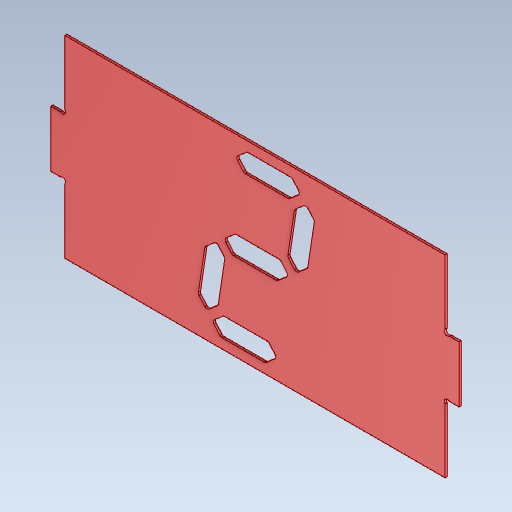
# Autodesk Inventor part: Cockpit_front_frame_cloth
Saved by Autodesk Inventor 2020 (Build 240168000, 168)
## iProperties
Created: 2022-04-24
Part Number: Cockpit_front_frame_cloth
Material: PET プラスチック
Document SubType Name: Modeling
Designer: Masato Kubotera
Density: 1.541 g/cm^3
Appearance: 滑らか - 赤
Description: PP T0.75
Author: Masato Kubotera
Autodesk Inventor part; units mm, degrees
ref_plane "YZ Plane" through (0, 0, 0) normal (1, 0, 0) x (0, 1, 0)
ref_plane "XZ Plane" through (0, 0, 0) normal (0, 1, 0) x (-1, 0, 0)
ref_plane "XY Plane" through (0, 0, 0) normal (0, 0, 1) x (1, 0, 0)
derived "Cockpit_front_frame.ipt"
sketch "スケッチ2" plane through (0, 0, 0) normal (0, 1, 0) x (-1, 0, 0)
  line L0 (-23.5, -22.5) -> (-28.5, -27.5)
  line L1 (-28.5, -27.5) -> (-28.5, -91)
  line L2 (-28.5, -91) -> (-23.5, -96)
  line L3 (-23.5, -96) -> (35.75, -96)
  line L4 (37.75, -98) -> (37.75, -131)
  line L5 (37.75, -131) -> (42.75, -136)
  line L6 (42.75, -136) -> (83.5, -136)
  line L7 (88.5, -131) -> (88.5, -20)
  line L8 (88.5, -20) -> (86, -17.5)
  line L9 (86, -17.5) -> (80.25, -17.5)
  line L10 (80.25, -17.5) -> (80.25, -22.5)
  line L11 (80.25, -22.5) -> (73.9849, -22.5)
  line L12 (72.5, -21.0151) -> (72.5, -17.5)
  line L13 (72.5, -17.5) -> (64.5, -17.5)
  line L14 (64.5, -17.5) -> (64.5, -21.0151)
  line L15 (63.0151, -22.5) -> (-23.5, -22.5)
  line L16 (-25.25, -25) -> (-20.25, -25) construction
  line L17 (-20.25, -25) -> (-20.25, -93.5) construction
  line L18 (-20.25, -93.5) -> (-25.25, -93.5) construction
  line L19 (-25.25, -93.5) -> (-25.25, -25) construction
  line L20 (-26, -25) -> (-25.25, -25) construction
  line L21 (-25.25, -93.5) -> (-26, -93.5) construction
  line L22 (-26, -93.5) -> (-26, -25) construction
  line L23 (-20.25, -93.5) -> (80.25, -93.5) construction
  line L24 (-20.25, -88.5) -> (80.25, -88.5) construction
  line L25 (80.25, -22.5) -> (80.25, -90.5) construction
  line L26 (80.25, -90.5) -> (85.25, -90.5) construction
  line L27 (85.25, -90.5) -> (85.25, -22.5) construction
  line L28 (80.25, -88.5) -> (80.25, -93.5) construction
  line L29 (80.25, -91) -> (85.25, -91) construction
  line L30 (85.25, -91) -> (85.25, -133.5) construction
  line L31 (80.25, -91) -> (80.25, -133.5) construction
  line L32 (80.25, -133.5) -> (85.25, -133.5) construction
  line L33 (40.25, -133.5) -> (40.25, -128.5) construction
  line L34 (40.25, -128.5) -> (40.25, -93.5) construction
  line L35 (45.25, -93.5) -> (45.25, -128.5) construction
  line L36 (40.25, -128.5) -> (45.25, -128.5) construction
  line L37 (42.75, -128.5) -> (42.75, -93.5) construction
  line L38 (40.25, -128.5) -> (79.1145, -128.5) construction
  line L39 (79.1145, -128.5) -> (79.1145, -133.5) construction
  line L40 (79.1145, -133.5) -> (40.25, -133.5) construction
  line L41 (40.25, -131) -> (79.1145, -131) construction
  line L42 (82.75, -91) -> (82.75, -133.5) construction
  circle A0 centre (82.75, -131) radius 2
  arc A1 (80.25, -128.5) -> (85.25, -128.5) centre (82.75, -131) ccw construction
  line L43 (80.25, -91) -> (-20.25, -91) construction
  line L44 (42.75, -111) -> (45.25, -111) construction
  line L45 (59.6822, -128.5) -> (59.6822, -131) construction
  line L46 (42.7, -115.5651) -> (42.7, -106.4349)
  line L47 (45.3, -107.05) -> (45.3, -114.95)
  line L48 (45.3, -117.05) -> (42.7, -104.95) construction
  line L49 (42.7, -117.05) -> (45.3, -104.95) construction
  line L50 (55.7322, -128.45) -> (63.6322, -128.45)
  line L51 (64.2473, -131.05) -> (55.1172, -131.05)
  line L52 (53.6322, -128.45) -> (65.7322, -131.05) construction
  line L53 (65.7322, -128.45) -> (53.6322, -131.05) construction
  line L54 (42.75, -105) -> (45.25, -105) construction
  line L55 (42.75, -117) -> (45.25, -117) construction
  arc A2 (44.1849, -104.95) -> (42.7, -106.4349) centre (43.4425, -105.6925) ccw
  arc A3 (45.3, -107.05) -> (45.3, -104.95) centre (45.3, -106) ccw
  arc A4 (42.7, -115.5651) -> (44.1849, -117.05) centre (43.4425, -116.3075) ccw
  arc A5 (45.3, -117.05) -> (45.3, -114.95) centre (45.3, -116) ccw
  line L56 (53.6822, -131) -> (53.6822, -128.5) construction
  line L57 (65.6822, -128.5) -> (65.6822, -131) construction
  arc A6 (53.6322, -129.5651) -> (55.1172, -131.05) centre (54.3747, -130.3075) ccw
  arc A7 (55.7322, -128.45) -> (53.6322, -128.45) centre (54.6822, -128.45) ccw
  arc A8 (64.2473, -131.05) -> (65.7322, -129.5651) centre (64.9898, -130.3075) ccw
  arc A9 (65.7322, -128.45) -> (63.6322, -128.45) centre (64.6822, -128.45) ccw
  line L58 (53.6322, -129.5651) -> (53.6322, -128.45)
  line L59 (65.7322, -128.45) -> (65.7322, -129.5651)
  line L60 (44.1849, -104.95) -> (45.3, -104.95)
  line L61 (45.3, -117.05) -> (44.1849, -117.05)
  circle A10 centre (47.6822, -131) radius 1.6
  line L62 (85.25, -22.5) -> (85.25, -17.5) construction
  line L63 (86, -17.5) -> (86, -90.5) construction
  line L64 (86, -90.5) -> (85.25, -90.5) construction
  line L65 (-18.5, -82.5) -> (-18.5, -61)
  arc A11 (-18.5, -82.5) -> (-16.5, -84.5) centre (-16.5, -82.5) ccw
  line L66 (45.5, -84.5) -> (-16.5, -84.5)
  arc A12 (45.5, -84.5) -> (47.5, -82.5) centre (45.5, -82.5) ccw
  line L67 (47.5, -61) -> (47.5, -82.5)
  arc A13 (47.5, -61) -> (45.5, -59) centre (45.5, -61) ccw
  line L68 (-16.5, -59) -> (45.5, -59)
  arc A14 (-16.5, -59) -> (-18.5, -61) centre (-16.5, -61) ccw
  line L69 (30, -88.5) -> (30, -91) construction
  line L70 (82.75, -22.5) -> (82.75, -90.5) construction
  circle A15 centre (82.75, -34) radius 1.6
  circle A16 centre (82.75, -34) radius 3
  circle A17 centre (82.75, -79) radius 1.6
  circle A18 centre (82.75, -79) radius 3
  line L71 (85.25, -22.5) -> (80.25, -22.5) construction
  arc A19 (85.25, -91) -> (80.25, -91) centre (82.75, -131) ccw construction
  circle A20 centre (47.6822, -131) radius 3
  circle A21 centre (42.75, -99) radius 1.6
  circle A22 centre (42.75, -99) radius 3
  line L72 (5, -88.5) -> (5, -91) construction
  line L73 (55, -88.5) -> (55, -91) construction
  line L74 (53.5651, -91.05) -> (6.4349, -91.05)
  line L75 (4.95, -89.5651) -> (4.95, -88.45)
  line L76 (7.05, -88.45) -> (52.95, -88.45)
  line L77 (55.05, -88.45) -> (55.05, -89.5651)
  line L78 (55.05, -91.05) -> (4.95, -88.45) construction
  line L79 (4.95, -91.05) -> (55.05, -88.45) construction
  arc A23 (7.05, -88.45) -> (4.95, -88.45) centre (6, -88.45) ccw
  arc A24 (4.95, -89.5651) -> (6.4349, -91.05) centre (5.6925, -90.3075) ccw
  arc A25 (55.05, -88.45) -> (52.95, -88.45) centre (54, -88.45) ccw
  arc A26 (53.5651, -91.05) -> (55.05, -89.5651) centre (54.3075, -90.3075) ccw
  line L80 (-20.25, -41) -> (80.25, -41) construction
  line L81 (80.25, -36) -> (-20.25, -36) construction
  line L82 (-20.25, -36) -> (-20.25, -41) construction
  line L83 (-20.25, -38.5) -> (80.25, -38.5) construction
  line L84 (30, -41) -> (30, -36) construction
  line L85 (53.5651, -35.95) -> (6.4349, -35.95)
  line L86 (6.4349, -41.05) -> (53.5651, -41.05)
  line L87 (55.05, -35.95) -> (4.95, -41.05) construction
  line L88 (4.95, -35.95) -> (55.5723, -41.1032) construction
  arc A27 (6.4349, -35.95) -> (4.95, -37.4349) centre (5.6925, -36.6925) ccw
  arc A28 (4.95, -39.5651) -> (6.4349, -41.05) centre (5.6925, -40.3075) ccw
  arc A29 (55.05, -37.4349) -> (53.5651, -35.95) centre (54.3075, -36.6925) ccw
  arc A30 (53.5651, -41.05) -> (55.05, -39.5651) centre (54.3075, -40.3075) ccw
  line L89 (5, -41) -> (5, -36) construction
  line L90 (55, -36) -> (55, -41) construction
  line L91 (4.95, -37.4349) -> (4.95, -39.5651)
  line L92 (55.05, -39.5651) -> (55.05, -37.4349)
  circle A31 centre (-2.5, -38.5) radius 1.6
  circle A32 centre (-2.5, -38.5) radius 3
  circle A33 centre (62.5, -38.5) radius 1.6
  circle A34 centre (62.5, -38.5) radius 3
  line L93 (-25.25, -44.25) -> (-22.75, -44.25) construction
  line L94 (-25.25, -49.25) -> (-26, -49.25) construction
  line L95 (-25.25, -74.25) -> (-22.75, -74.25) construction
  line L96 (-25.25, -69.25) -> (-26, -69.25) construction
  line L97 (-26, -59.25) -> (-25.25, -59.25) construction
  line L98 (-25.25, -59.25) -> (-22.75, -59.25) construction
  line L99 (-22.75, -25) -> (-22.75, -93.5) construction
  arc A35 (63.0151, -22.5) -> (64.5, -21.0151) centre (63.7575, -21.7575) ccw
  arc A36 (72.5, -21.0151) -> (73.9849, -22.5) centre (73.2425, -21.7575) ccw
  line L100 (56.75, -22.5) -> (56.75, -32.5) construction
  line L101 (56.75, -32.5) -> (80.25, -32.5) construction
  line L102 (80.25, -32.5) -> (80.25, -22.5) construction
  line L103 (68.5, -17.5) -> (68.5, -32.5) construction
  line L104 (60.5, -22.5) -> (60.5, -17.5) construction
  line L105 (76.5, -22.5) -> (76.5, -17.5) construction
  line L106 (-22.7, -46.3) -> (-22.7, -72.2)
  line L107 (-25.3, -72.8151) -> (-25.3, -69.564)
  line L108 (-25.3, -44.2) -> (-22.7, -74.3) construction
  line L109 (-22.7, -44.2) -> (-25.3, -74.3) construction
  arc A37 (-22.7, -46.3) -> (-22.7, -44.2) centre (-22.7, -45.25) ccw
  arc A38 (-23.8151, -44.2) -> (-25.3, -45.6849) centre (-24.5575, -44.9425) ccw
  line L110 (-23.8151, -44.2) -> (-22.7, -44.2)
  arc A39 (-22.7, -74.3) -> (-22.7, -72.2) centre (-22.7, -73.25) ccw
  arc A40 (-25.3, -72.8151) -> (-23.8151, -74.3) centre (-24.5575, -73.5575) ccw
  line L111 (-22.7, -74.3) -> (-23.8151, -74.3)
  line L112 (-26.3, -49.9848) -> (-26.3, -68.5152)
  arc A41 (-26.3, -68.5152) -> (-25.3, -69.564) centre (-25.25, -68.5152) ccw
  arc A42 (-25.3, -48.936) -> (-26.3, -49.9848) centre (-25.25, -49.9848) ccw
  line L113 (-25.3, -48.936) -> (-25.3, -45.6849)
  circle A43 centre (-22.75, -36.75) radius 1.6
  circle A44 centre (-22.75, -36.75) radius 3
  circle A45 centre (-22.75, -81.75) radius 1.6
  circle A46 centre (-22.75, -81.75) radius 3
  line L114 (64.5, -22.5) -> (72.5, -22.5)
  line L115 (85.25, -17.5) -> (52.5, -17.5) construction
  line L116 (52.5, -17.5) -> (52.5, -22.5) construction
  circle A47 centre (82.75, -93.5) radius 1.475
  circle A48 centre (82.75, -98.5) radius 1.475
  circle A49 centre (82.75, -103.5) radius 1.475
  line L117 (49.75, -93.5) -> (78.25, -93.5)
  line L118 (80.25, -95.5) -> (80.25, -124)
  line L119 (78.25, -126) -> (49.75, -126)
  line L120 (47.75, -124) -> (47.75, -95.5)
  arc A50 (49.75, -93.5) -> (47.75, -95.5) centre (49.75, -95.5) ccw
  arc A51 (47.75, -124) -> (49.75, -126) centre (49.75, -124) ccw
  arc A52 (78.25, -126) -> (80.25, -124) centre (78.25, -124) ccw
  arc A53 (80.25, -95.5) -> (78.25, -93.5) centre (78.25, -95.5) ccw
  arc A54 (37.75, -98) -> (35.75, -96) centre (35.75, -98) ccw
  circle A55 centre (-13.5, -55) radius 1.75
  circle A56 centre (-13.5, -55) radius 2
  line L121 (74.85, -78.65) -> (65.65, -78.65) construction
  line L122 (65.65, -78.65) -> (65.65, -64.85) construction
  line L123 (65.65, -64.85) -> (74.85, -64.85) construction
  line L124 (74.85, -64.85) -> (74.85, -78.65) construction
  line L125 (74.85, -78.65) -> (65.65, -64.85) construction
  line L126 (65.65, -78.65) -> (74.85, -64.85) construction
  line L127 (64.95, -64.2) -> (75.55, -64.2) construction
  line L128 (75.55, -64.2) -> (75.55, -79.3) construction
  line L129 (75.55, -79.3) -> (64.95, -79.3) construction
  line L130 (64.95, -79.3) -> (64.95, -64.2) construction
  line L131 (64.95, -64.2) -> (75.55, -79.3) construction
  line L132 (75.55, -64.2) -> (64.95, -79.3) construction
  line L133 (66.3849, -64.15) -> (74.1151, -64.15)
  line L134 (75.6, -65.6349) -> (75.6, -77.8651)
  line L135 (75.6, -79.35) -> (64.9, -64.15) construction
  line L136 (64.9, -79.35) -> (75.6, -64.15) construction
  line L137 (74.9, -78.7) -> (65.6, -64.8) construction
  line L138 (65.6, -78.7) -> (74.9, -64.8) construction
  arc A57 (66.3849, -64.15) -> (64.9, -65.6349) centre (65.6425, -64.8925) ccw
  arc A58 (67.0849, -64.8) -> (65.6, -66.2849) centre (66.3425, -65.5425) ccw
  line L139 (64.9, -71.75) -> (75.6, -71.75) construction
  line L140 (70.25, -64.15) -> (70.25, -78.7063) construction
  arc A59 (75.6, -65.6349) -> (74.1151, -64.15) centre (74.8575, -64.8925) ccw
  arc A60 (74.9, -66.2849) -> (73.4151, -64.8) centre (74.1575, -65.5425) ccw
  arc A61 (64.9, -77.8651) -> (66.3849, -79.35) centre (65.6425, -78.6075) ccw
  arc A62 (65.6, -77.2151) -> (67.0849, -78.7) centre (66.3425, -77.9575) ccw
  arc A63 (74.1151, -79.35) -> (75.6, -77.8651) centre (74.8575, -78.6075) ccw
  arc A64 (73.4151, -78.7) -> (74.9, -77.2151) centre (74.1575, -77.9575) ccw
  line L141 (67.0849, -64.8) -> (73.4151, -64.8)
  line L142 (74.9, -66.2849) -> (74.9, -77.2151)
  line L143 (64.9, -77.8651) -> (64.9, -65.6349)
  line L144 (65.6, -77.2151) -> (65.6, -66.2849)
  line L145 (73.4151, -78.7) -> (67.0849, -78.7)
  line L146 (74.1151, -79.35) -> (66.3849, -79.35)
  line L147 (-18.5, -71.75) -> (47.5, -71.75) construction
  line L148 (82.75, -56.5) -> (85.25, -56.5) construction
  line L149 (86, -54) -> (85.25, -54) construction
  line L150 (82.7, -69.45) -> (82.7, -43.55)
  line L151 (85.3057, -71.616) -> (82.7, -41.45) construction
  line L152 (82.7, -71.55) -> (85.3, -41.45) construction
  arc A65 (82.7, -41.45) -> (82.7, -43.55) centre (82.7, -42.5) ccw
  arc A66 (85.3, -42.9349) -> (83.8151, -41.45) centre (84.5575, -42.1925) ccw
  arc A67 (82.7, -69.45) -> (82.7, -71.55) centre (82.7, -70.5) ccw
  arc A68 (83.8151, -71.55) -> (85.3, -70.0651) centre (84.5575, -70.8075) ccw
  line L153 (82.75, -41.5) -> (85.25, -41.5) construction
  line L154 (82.75, -71.5) -> (85.25, -71.5) construction
  arc A69 (86.25, -47.1801) -> (85.3, -46.1348) centre (85.2, -47.1801) ccw
  line L155 (86.25, -47.1801) -> (86.25, -65.8199)
  line L156 (85.25, -46.5) -> (86, -46.5) construction
  line L157 (85.25, -66.5) -> (86, -66.5) construction
  arc A70 (85.3, -66.8652) -> (86.25, -65.8199) centre (85.2, -65.8199) ccw
  line L158 (85.3, -42.9349) -> (85.3, -46.1348)
  line L159 (85.3, -66.8652) -> (85.3, -70.0651)
  line L160 (83.8151, -71.55) -> (82.7, -71.55)
  line L161 (82.7, -41.45) -> (83.8151, -41.45)
  line L162 (83.5, -136) -> (88.5, -131)
  point P0 (0, 0)
  point P1 (-25.7227, -96)
  point P2 (-23.5, -22.5)
  point P3 (44, -111)
  point P4 (59.6822, -129.75)
  point P5 (30, -89.75)
  point P6 (30, -38.5)
  point P7 (4.95, -41.05)
  point P8 (52.5, -22)
  point P9 (-24, -59.25)
  point P10 (70.25, -71.75)
  point P11 (70.25, -71.75)
  point P12 (84, -56.5)
  dimension "d4" = 0.75
  measures "d4" distance of L20.start L20.end
sketch "スケッチ3" plane through (25.25, 0, 0) normal (1, 0, 0) x (0, 1, 0)
  line L0 (-135, -25) -> (0, -25)
  line L1 (0, -93.5) -> (-135, -93.5)
  line L2 (1.4849, -44.25) -> (5, -44.25)
  line L3 (5, -44.25) -> (5, -74.25)
  line L4 (0, -59.25) -> (-135, -59.25) construction
  arc A0 (0, -42.7651) -> (1.4849, -44.25) centre (0.7425, -43.5075) ccw
  line L5 (0, -25) -> (0, -42.7651)
  arc A1 (1.4849, -74.25) -> (0, -75.7349) centre (0.7425, -74.9925) ccw
  line L6 (1.4849, -74.25) -> (5, -74.25)
  line L7 (0, -44.25) -> (0, -74.25)
  line L8 (0, -75.7349) -> (0, -93.5)
  line L9 (-67.5, -25) -> (-67.5, -93.5) construction
  line L10 (-136.4849, -74.25) -> (-140, -74.25)
  arc A2 (-135, -75.7349) -> (-136.4849, -74.25) centre (-135.7425, -74.9925) ccw
  line L11 (-136.4849, -44.25) -> (-140, -44.25)
  line L12 (-140, -44.25) -> (-140, -74.25)
  line L13 (-135, -75.7349) -> (-135, -93.5)
  arc A3 (-136.4849, -44.25) -> (-135, -42.7651) centre (-135.7425, -43.5075) ccw
  line L14 (-135, -44.25) -> (-135, -74.25)
  line L15 (-135, -25) -> (-135, -42.7651)
  line L16 (-7, -30) -> (-128, -30)
  line L17 (-130, -32) -> (-130, -34)
  line L18 (-128, -36) -> (-7, -36)
  line L19 (-5, -34) -> (-5, -32)
  line L20 (-5, -30) -> (-130, -36) construction
  line L21 (-130, -30) -> (-5, -36) construction
  line L22 (-7, -88.5) -> (-128, -88.5)
  line L23 (-130, -86.5) -> (-130, -43)
  line L24 (-128, -41) -> (-7, -41)
  line L25 (-5, -43) -> (-5, -86.5)
  line L26 (-5, -88.5) -> (-130, -41) construction
  line L27 (-130, -88.5) -> (-5, -41) construction
  arc A4 (-128, -30) -> (-130, -32) centre (-128, -32) ccw
  arc A5 (-130, -34) -> (-128, -36) centre (-128, -34) ccw
  arc A6 (-7, -36) -> (-5, -34) centre (-7, -34) ccw
  arc A7 (-5, -32) -> (-7, -30) centre (-7, -32) ccw
  arc A8 (-5, -43) -> (-7, -41) centre (-7, -43) ccw
  arc A9 (-128, -41) -> (-130, -43) centre (-128, -43) ccw
  arc A10 (-130, -86.5) -> (-128, -88.5) centre (-128, -86.5) ccw
  arc A11 (-7, -88.5) -> (-5, -86.5) centre (-7, -86.5) ccw
  point P0 (0, 0)
  point P1 (0, -93.5)
  point P2 (-135, -93.5)
  point P3 (-135, -25)
  point P4 (-67.5, -33)
  point P5 (-67.5, -64.75)
  point P6 (0, -36)
  point P7 (0, -36)
  point P8 (0, -36)
  point P9 (0, -41)
  point P10 (0, -41)
  point P11 (0, -41)
ref_plane "作業平面1" through (25.25, -135, -25) normal (-1, 0, 0) x (0, 1, 0)
sketch "スケッチ4" plane through (25.25, -135, -25) normal (-1, 0, 0) x (0, 1, 0)
  arc A0 (136.4849, 24.25) -> (135, 22.7651) centre (135.7425, 23.5075) ccw
  line L0 (136.4849, 24.25) -> (140, 24.25)
  line L1 (140, 24.25) -> (140, 44.25)
  line L2 (135, 19.25) -> (135, 49.25) construction
  line L3 (140, 19.25) -> (140, 49.25) construction
  line L4 (135, 34.25) -> (0, 34.25) construction
  line L5 (67.5, 0) -> (67.5, 68.5) construction
  line L6 (0, 0) -> (135, 0) projected
  line L7 (135, 68.5) -> (0, 68.5) projected
  arc A1 (135, 45.7349) -> (136.4849, 44.25) centre (135.7425, 44.9925) ccw
  line L8 (136.4849, 44.25) -> (140, 44.25)
  line L9 (135, 22.7651) -> (135, 0)
  line L10 (135, 45.7349) -> (135, 68.5)
  arc A2 (0, 22.7651) -> (-1.4849, 24.25) centre (-0.7425, 23.5075) ccw
  line L11 (-1.4849, 24.25) -> (-5, 24.25)
  line L12 (-1.4849, 44.25) -> (-5, 44.25)
  arc A3 (-1.4849, 44.25) -> (0, 45.7349) centre (-0.7425, 44.9925) ccw
  line L13 (0, 22.7651) -> (0, 0)
  line L14 (0, 45.7349) -> (0, 68.5)
  line L15 (-5, 24.25) -> (-5, 44.25)
  line L16 (51.1141, 58.6095) -> (54.1517, 56.0021)
  line L17 (53.0682, 60.8859) -> (56.1057, 58.2784)
  line L18 (55.0145, 64.6885) -> (52.9607, 62.296)
  line L19 (49.704, 58.5021) -> (47.6502, 56.1095)
  line L20 (55.7733, 65.0372) -> (70.8617, 65.0372)
  line L21 (72.6043, 58.3859) -> (74.658, 60.7784)
  line L22 (71.513, 64.796) -> (74.5506, 62.1885)
  line L23 (56.7571, 58.0372) -> (71.8455, 58.0372)
  line L24 (54.4888, 55.3948) -> (56.7748, 40.4805)
  line L25 (56.5452, 39.6777) -> (54.4914, 37.2851)
  line L26 (53.0813, 37.1777) -> (50.0437, 39.7851)
  line L27 (47.4206, 55.3066) -> (49.7066, 40.3924)
  line L28 (50.3553, 59.2608) -> (53.84, 36.5264) construction
  line L29 (75.3094, 61.5372) -> (52.3094, 61.5372) construction
  arc A4 (51.1141, 58.6095) -> (49.704, 58.5021) centre (50.4628, 57.8507) ccw
  arc A5 (54.4888, 55.3948) -> (54.1517, 56.0021) centre (53.5003, 55.2433) ccw
  arc A6 (56.5452, 39.6777) -> (56.7748, 40.4805) centre (55.7864, 40.329) ccw
  arc A7 (53.0813, 37.1777) -> (54.4914, 37.2851) centre (53.7326, 37.9365) ccw
  arc A8 (49.7066, 40.3924) -> (50.0437, 39.7851) centre (50.695, 40.5439) ccw
  arc A9 (47.6502, 56.1095) -> (47.4206, 55.3066) centre (48.409, 55.4582) ccw
  arc A10 (71.8455, 58.0372) -> (72.6043, 58.3859) centre (71.8455, 59.0372) ccw
  arc A11 (74.658, 60.7784) -> (74.5506, 62.1885) centre (73.8992, 61.4298) ccw
  arc A12 (71.513, 64.796) -> (70.8617, 65.0372) centre (70.8617, 64.0372) ccw
  arc A13 (55.7733, 65.0372) -> (55.0145, 64.6885) centre (55.7733, 64.0372) ccw
  arc A14 (52.9607, 62.296) -> (53.0682, 60.8859) centre (53.7195, 61.6446) ccw
  arc A15 (56.1057, 58.2784) -> (56.7571, 58.0372) centre (56.7571, 59.0372) ccw
  line L30 (78.72, 58.6095) -> (81.7576, 56.0021)
  line L31 (77.3099, 58.5021) -> (75.2561, 56.1095)
  arc A16 (78.72, 58.6095) -> (77.3099, 58.5021) centre (78.0687, 57.8507) ccw
  line L32 (75.0264, 55.3066) -> (77.3125, 40.3924)
  arc A17 (75.2561, 56.1095) -> (75.0264, 55.3066) centre (76.0149, 55.4582) ccw
  arc A18 (82.0947, 55.3948) -> (81.7576, 56.0021) centre (81.1062, 55.2433) ccw
  line L33 (82.0947, 55.3948) -> (84.3807, 40.4805)
  arc A19 (84.151, 39.6777) -> (84.3807, 40.4805) centre (83.3922, 40.329) ccw
  line L34 (84.151, 39.6777) -> (82.0973, 37.2851)
  arc A20 (80.6871, 37.1777) -> (82.0973, 37.2851) centre (81.3385, 37.9365) ccw
  line L35 (80.6871, 37.1777) -> (77.6496, 39.7851)
  arc A21 (77.3125, 40.3924) -> (77.6496, 39.7851) centre (78.3009, 40.5439) ccw
  line L36 (55.2967, 31.3223) -> (58.3342, 28.7149)
  line L37 (53.8865, 31.2149) -> (51.8328, 28.8223)
  arc A22 (55.2967, 31.3223) -> (53.8865, 31.2149) centre (54.6453, 30.5635) ccw
  line L38 (51.6031, 28.0195) -> (53.8891, 13.1052)
  arc A23 (51.8328, 28.8223) -> (51.6031, 28.0195) centre (52.5915, 28.171) ccw
  arc A24 (58.6713, 28.1076) -> (58.3342, 28.7149) centre (57.6829, 27.9561) ccw
  line L39 (58.6713, 28.1076) -> (60.9573, 13.1934)
  arc A25 (60.7277, 12.3905) -> (60.9573, 13.1934) centre (59.9689, 13.0418) ccw
  line L40 (60.7277, 12.3905) -> (58.6739, 9.9979)
  arc A26 (57.2638, 9.8905) -> (58.6739, 9.9979) centre (57.9151, 10.6493) ccw
  line L41 (57.2638, 9.8905) -> (54.2262, 12.4979)
  arc A27 (53.8891, 13.1052) -> (54.2262, 12.4979) centre (54.8776, 13.2567) ccw
  line L42 (82.9025, 31.3223) -> (85.9401, 28.7149)
  line L43 (81.4924, 31.2149) -> (79.4386, 28.8223)
  arc A28 (82.9025, 31.3223) -> (81.4924, 31.2149) centre (82.2512, 30.5635) ccw
  line L44 (79.209, 28.0195) -> (81.495, 13.1052)
  arc A29 (79.4386, 28.8223) -> (79.209, 28.0195) centre (80.1974, 28.171) ccw
  arc A30 (86.2772, 28.1076) -> (85.9401, 28.7149) centre (85.2887, 27.9561) ccw
  line L45 (86.2772, 28.1076) -> (88.5632, 13.1934)
  arc A31 (88.3336, 12.3905) -> (88.5632, 13.1934) centre (87.5748, 13.0418) ccw
  line L46 (88.3336, 12.3905) -> (86.2798, 9.9979)
  arc A32 (84.8697, 9.8905) -> (86.2798, 9.9979) centre (85.521, 10.6493) ccw
  line L47 (84.8697, 9.8905) -> (81.8321, 12.4979)
  arc A33 (81.495, 13.1052) -> (81.8321, 12.4979) centre (82.4834, 13.2567) ccw
  line L48 (59.9558, 37.75) -> (75.0442, 37.75)
  arc A34 (59.9558, 37.75) -> (59.197, 37.4013) centre (59.9558, 36.75) ccw
  line L49 (59.197, 37.4013) -> (57.1432, 35.0088)
  arc A35 (57.1432, 35.0088) -> (57.2507, 33.5987) centre (57.902, 34.3574) ccw
  line L50 (57.2507, 33.5987) -> (60.2882, 30.9912)
  arc A36 (60.2882, 30.9912) -> (60.9396, 30.75) centre (60.9396, 31.75) ccw
  line L51 (60.9396, 30.75) -> (76.028, 30.75)
  arc A37 (76.028, 30.75) -> (76.7868, 31.0987) centre (76.028, 31.75) ccw
  line L52 (76.7868, 31.0987) -> (78.8406, 33.4912)
  arc A38 (78.8406, 33.4912) -> (78.7331, 34.9013) centre (78.0818, 34.1426) ccw
  line L53 (75.6955, 37.5088) -> (78.7331, 34.9013)
  arc A39 (75.6955, 37.5088) -> (75.0442, 37.75) centre (75.0442, 36.75) ccw
  line L54 (64.1383, 10.4628) -> (79.2267, 10.4628)
  arc A40 (64.1383, 10.4628) -> (63.3795, 10.1141) centre (64.1383, 9.4628) ccw
  line L55 (63.3795, 10.1141) -> (61.3258, 7.7216)
  arc A41 (61.3258, 7.7216) -> (61.4332, 6.3115) centre (62.0845, 7.0702) ccw
  line L56 (61.4332, 6.3115) -> (64.4708, 3.704)
  arc A42 (64.4708, 3.704) -> (65.1221, 3.4628) centre (65.1221, 4.4628) ccw
  line L57 (65.1221, 3.4628) -> (80.2105, 3.4628)
  arc A43 (80.2105, 3.4628) -> (80.9693, 3.8115) centre (80.2105, 4.4628) ccw
  line L58 (80.9693, 3.8115) -> (83.0231, 6.204)
  arc A44 (83.0231, 6.204) -> (82.9156, 7.6141) centre (82.2643, 6.8554) ccw
  line L59 (79.8781, 10.2216) -> (82.9156, 7.6141)
  arc A45 (79.8781, 10.2216) -> (79.2267, 10.4628) centre (79.2267, 9.4628) ccw
  line L60 (67.5, 37.75) -> (68.4838, 30.75) construction
  point P0 (135, -25)
  point P1 (135, 24.25)
  point P2 (135, 24.25)
  point P3 (135, 24.25)
  point P4 (135, 24.25)
  point P5 (47.3509, 55.7608)
  point P6 (54.4327, 55.7608)
  point P7 (56.3867, 58.0372)
  point P8 (55.3138, 65.0372)
  point P9 (71.232, 65.0372)
  point P10 (72.305, 58.0372)
  point P11 (56.8444, 40.0264)
  point P12 (49.7627, 40.0264)
  point P13 (77.9612, 59.2608)
  point P14 (82.0386, 55.7608)
  point P15 (74.9568, 55.7608)
  point P16 (77.3686, 40.0264)
  point P17 (84.4503, 40.0264)
  point P18 (81.4459, 36.5264)
  point P19 (54.5379, 31.9736)
  point P20 (58.6152, 28.4736)
  point P21 (51.5335, 28.4736)
  point P22 (53.9452, 12.7392)
  point P23 (61.027, 12.7392)
  point P24 (58.0226, 9.2392)
  point P25 (82.1437, 31.9736)
  point P26 (86.2211, 28.4736)
  point P27 (79.1393, 28.4736)
  point P28 (81.5511, 12.7392)
  point P29 (88.6328, 12.7392)
  point P30 (85.6284, 9.2392)
  point P31 (75.4145, 37.75)
  point P32 (59.4963, 37.75)
  point P33 (56.4919, 34.25)
  point P34 (60.5692, 30.75)
  point P35 (76.4875, 30.75)
  point P36 (79.4919, 34.25)
  point P37 (79.5971, 10.4628)
  point P38 (63.6788, 10.4628)
  point P39 (60.6744, 6.9628)
  point P40 (64.7518, 3.4628)
  point P41 (80.67, 3.4628)
  point P42 (83.6744, 6.9628)
  dimension "d1" = 1.05
  dimension "d13" = 3
  dimension "d14" = 7
  dimension "d15" = 7
  dimension "d16" = 23
  dimension "d17" = 23
  dimension "d18" = 1
  dimension "d19" = 1
  dimension "d20" = 27.6059
  dimension "d21" = 27.6059
  dimension "d22" = 27.6059
  dimension "d25" = 8
  constraints: 110 end point, 93 point on circle, 89 point on line, 46 centre point, 24 tangent, 12 symmetric about line, 10 equal radius, 7 collinear, 6 parallel, 2 horizontal, 2 midpoint, 2 perpendicular, 1 vertical, 190 other
  measures "d1" radius of A0
  measures "d13" distance between parallel lines of L16 L17
  measures "d14" distance between parallel lines of L23 L20
  measures "d15" distance between parallel lines of L24 L27
  measures "d16" distance of L29.start L29.end
  measures "d17" distance of L28.start L28.end
  measures "d18" radius of A4
  measures "d19" radius of A10
  measures "d20" distance of L16.start L30.start
  measures "d21" distance of L16.start L36.start
  measures "d22" distance of L20.start L48.start
  measures "d25" angle of L5 L60
extrude "押し出し1" add sketch "スケッチ4" against normal blind 0.75 contours A0 L9 L6 L13 A2 L11 L15 L12 A3 L14 L7 L10 A1 L8 L1 L0 | L30 A18 L33 A19 L34 A20 L35 A21 L32 A17 L31 A16 | L36 A24 L39 A25 L40 A26 L41 A27 L38 A23 L37 A22
equation "\"d15\" = d14"
equation "\"d17\" = d16"
equation "\"d2\" = d4"
